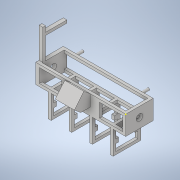
# Autodesk Inventor part: Diff housing
Saved by Autodesk Inventor 2021 (Build 250183000, 183)
## iProperties
Created: 2020-10-15
Part Number: Diff housing
Material: Generic
Document SubType Name: Modeling
Designer: nabee
Density: 1 g/cm^3
Appearance: Default
Author: nabee
Autodesk Inventor part; units mm, degrees
ref_plane "YZ Plane" through (0, 0, 0) normal (1, 0, 0) x (0, 1, 0)
ref_plane "XZ Plane" through (0, 0, 0) normal (0, 1, 0) x (-1, 0, 0)
sketch "Sketch1" plane through (0, 0, 0) normal (0, 0, 1) x (1, 0, 0)
  line L0 (0, 0) -> (500, 0)
  line L1 (500, 0) -> (500, 140)
  line L2 (500, 140) -> (0, 140)
  line L3 (0, 140) -> (0, 0)
  dimension "d0" = 140
  dimension "d1" = 500
  constraints: 8 end point, 2 parallel, 1 horizontal, 1 perpendicular
  measures "d0" distance of L2.end L0.start
  measures "d1" distance of L0.start L0.end
extrude "Extrusion1" add sketch "Sketch1" along normal blind 200
sketch "Sketch2" plane through (0, 140, 0) normal (0, 1, 0) x (1, 0, 0)
  line L0 (20, -20) -> (480, -20)
  line L1 (480, -20) -> (480, -180)
  line L2 (480, -180) -> (20, -180)
  line L3 (20, -180) -> (20, -20)
  line L4 (500, 0) -> (0, 0) projected
  line L5 (0, 0) -> (0, -200) projected
  line L6 (500, -200) -> (0, -200) projected
  line L7 (500, 0) -> (500, -200) projected
  dimension "d4" = 20
  dimension "d5" = 20
  dimension "d6" = 20
  dimension "d7" = 20
  constraints: 8 end point, 2 parallel, 1 horizontal, 1 perpendicular
  measures "d4" distance between parallel lines of L4 L0
  measures "d5" distance between parallel lines of L5 L3
  measures "d6" distance between parallel lines of L6 L2
  measures "d7" distance between parallel lines of L7 L1
extrude "Extrusion2" cut sketch "Sketch2" against normal blind 200 contours L0 L1 L2 L3
sketch "Sketch3" plane through (0, 0, 200) normal (0, 0, 1) x (1, 0, 0)
  line L0 (20, 120) -> (480, 120)
  line L1 (480, 120) -> (480, 20)
  line L2 (480, 20) -> (20, 20)
  line L3 (20, 20) -> (20, 120)
  line L4 (500, 140) -> (0, 140) projected
  line L5 (0, 140) -> (0, 0) projected
  line L6 (0, 0) -> (500, 0) projected
  line L7 (500, 0) -> (500, 140) projected
  dimension "d10" = 20
  dimension "d11" = 20
  dimension "d12" = 20
  dimension "d13" = 20
  constraints: 8 end point, 2 parallel, 1 horizontal, 1 perpendicular
  measures "d10" distance between parallel lines of L4 L0
  measures "d11" distance between parallel lines of L5 L3
  measures "d12" distance between parallel lines of L6 L2
  measures "d13" distance between parallel lines of L7 L1
extrude "Extrusion3" cut sketch "Sketch3" against normal blind 200 contours L0 L1 L2 L3
sketch "Sketch4" plane through (500, 0, 0) normal (1, 0, 0) x (0, 0, -1)
  line L0 (0, 140) -> (-200, 140) projected
  circle A0 centre (-100, 70) radius 23.813
  point P0 (0, 0)
  dimension "d16" = 47.626
  constraints: 1 centre point
  measures "d16" diameter of A0
extrude "Extrusion4" cut sketch "Sketch4" against normal blind 900
sketch "Sketch5" plane through (500, 0, 0) normal (1, 0, 0) x (0, 0, -1)
  line L0 (0, 140) -> (-200, 140) projected
  line L1 (-200, 140) -> (0, 140)
  line L2 (0, 140) -> (0, 0)
  line L3 (0, 0) -> (-200, 0)
  line L4 (-200, 0) -> (-200, 140)
  constraints: 8 end point, 2 parallel, 1 horizontal, 1 perpendicular
extrude "Extrusion5" add sketch "Sketch5" along normal blind 146.467
sketch "Sketch7" plane through (646.467, 0, 0) normal (1, 0, 0) x (0, 0, -1)
  circle A0 centre (-100, 70) radius 23.813 projected
  circle A1 centre (-100, 70) radius 23.813
  point P0 (0, 0)
  constraints: 1 centre point, 1 coincident
extrude "Extrusion6" cut sketch "Sketch7" against normal blind 146.467
sketch "Sketch8" plane through (0, 0, 200) normal (0, 0, 1) x (1, 0, 0)
  line L0 (20, 120) -> (480, 120) projected
  line L1 (480, 120) -> (626.467, 120)
  line L2 (626.467, 120) -> (626.467, 20)
  line L3 (626.467, 20) -> (480, 20)
  line L4 (480, 20) -> (480, 120)
  line L5 (646.467, 140) -> (646.467, 0) projected
  point P0 (0, 0)
  dimension "d27" = 20
  constraints: 8 end point, 2 parallel, 1 horizontal, 1 perpendicular
  measures "d27" distance between parallel lines of L5 L2
extrude "Extrusion7" cut sketch "Sketch8" against normal blind 600
sketch "Sketch9" plane through (0, 140, 200) normal (0, 1, 0) x (1, 0, 0)
  line L0 (480, 180) -> (20, 180) projected
  line L1 (480, 180) -> (626.467, 180)
  line L2 (626.467, 180) -> (626.467, 20)
  line L3 (626.467, 20) -> (480, 20)
  line L4 (480, 20) -> (480, 180)
  line L5 (646.467, 200) -> (646.467, 0) projected
  point P0 (0, 200)
  dimension "d30" = 20
  constraints: 8 end point, 2 parallel, 1 horizontal, 1 perpendicular
  measures "d30" distance between parallel lines of L5 L2
extrude "Extrusion8" cut sketch "Sketch9" against normal blind 600
sketch "Sketch10" plane through (646.467, 0, 0) normal (1, 0, 0) x (0, 0, -1)
  line L0 (-200, 140) -> (0, 140)
  line L1 (0, 140) -> (0, 0)
  line L2 (0, 0) -> (-200, 0)
  line L3 (-200, 0) -> (-200, 140)
  constraints: 8 end point, 2 parallel, 1 horizontal, 1 perpendicular
extrude "Extrusion9" add sketch "Sketch10" along normal blind 10
sketch "Sketch11" plane through (656.467, 0, 0) normal (1, 0, 0) x (0, 0, -1)
  line L0 (0, 140) -> (-200, 140) projected
  line L1 (0, 140) -> (0, 0) projected
  line L2 (-200, 140) -> (0, 140)
  line L3 (0, 140) -> (0, 0)
  line L4 (0, 0) -> (-200, 0)
  line L5 (-200, 0) -> (-200, 140)
  constraints: 8 end point, 2 parallel, 1 horizontal, 1 perpendicular
extrude "Extrusion10" cut sketch "Sketch11" against normal blind 3.764
sketch "Sketch12" plane through (652.703, 0, 0) normal (1, 0, 0) x (0, 0, -1)
  circle A0 centre (-100, 70) radius 23.813 projected
  circle A1 centre (-100, 70) radius 23.813
  point P0 (0, 0)
  constraints: 1 centre point, 1 coincident
extrude "Extrusion11" cut sketch "Sketch12" against normal blind 200
sketch "Sketch14" plane through (0, 0, 200) normal (0, 0, 1) x (1, 0, 0)
  line L0 (652.703, 140) -> (452.703, 140)
  line L1 (452.703, 140) -> (452.703, 0)
  line L2 (652.703, 0) -> (652.703, 140)
  line L3 (0, 0) -> (652.703, 0) projected
  line L4 (652.703, 0) -> (652.703, -140)
  line L5 (652.703, -140) -> (452.703, -140)
  line L6 (452.703, -140) -> (452.703, 0)
  dimension "d47" = 200
  dimension "d48" = 140
  constraints: 12 end point, 3 perpendicular, 1 horizontal, 1 parallel, 1 vertical
  measures "d47" distance of L0.start L0.end
  measures "d48" distance of L2.start L4.end
extrude "Extrusion13" add sketch "Sketch14" along normal blind 160
sketch "Sketch15" plane through (0, 0, 360) normal (0, 0, 1) x (1, 0, 0)
  line L0 (632.703, -120) -> (472.703, -120)
  line L1 (472.703, -120) -> (472.703, 120)
  line L2 (472.703, 120) -> (632.703, 120)
  line L3 (632.703, 120) -> (632.703, -120)
  line L4 (452.703, -140) -> (652.703, -140) projected
  line L5 (652.703, -140) -> (652.703, 140) projected
  line L6 (652.703, 140) -> (452.703, 140) projected
  line L7 (452.703, 140) -> (452.703, -140) projected
  point P0 (0, 0)
  dimension "d51" = 20
  dimension "d52" = 20
  dimension "d53" = 20
  dimension "d54" = 20
  constraints: 8 end point, 2 parallel, 1 horizontal, 1 perpendicular
  measures "d51" distance between parallel lines of L4 L0
  measures "d52" distance between parallel lines of L5 L3
  measures "d53" distance between parallel lines of L6 L2
  measures "d54" distance between parallel lines of L7 L1
extrude "Extrusion14" cut sketch "Sketch15" against normal blind 160 contours L0 L1 L2 L3
sketch "Sketch16" plane through (452.703, -140, 200) normal (-1, 0, 0) x (0, 0, 1)
  line L0 (140, 20) -> (20, 20)
  line L1 (20, 20) -> (20, 260)
  line L2 (20, 260) -> (140, 260)
  line L3 (140, 260) -> (140, 20)
  line L4 (0, 0) -> (160, 0) projected
  line L5 (160, 280) -> (160, 0) projected
  line L6 (0, 140) -> (0, 0) projected
  line L7 (0, 280) -> (160, 280) projected
  point P0 (-200, 140)
  dimension "d57" = 20
  dimension "d58" = 20
  dimension "d59" = 20
  dimension "d60" = 20
  constraints: 8 end point, 2 parallel, 1 horizontal, 1 perpendicular
  measures "d57" distance between parallel lines of L4 L0
  measures "d58" distance between parallel lines of L5 L3
  measures "d59" distance between parallel lines of L6 L1
  measures "d60" distance between parallel lines of L7 L2
extrude "Extrusion15" cut sketch "Sketch16" against normal blind 900
sketch "Sketch17" plane through (452.703, -140, 200) normal (0, -1, 0) x (1, 0, 0)
  line L0 (180, 160) -> (180, 140) projected
  line L1 (20, 20) -> (20, 0) projected
  line L2 (180, 140) -> (20, 140)
  line L3 (20, 140) -> (20, 20)
  line L4 (20, 20) -> (180, 20)
  line L5 (180, 20) -> (180, 140)
  point P0 (-452.703, -200)
  constraints: 8 end point, 2 parallel, 1 horizontal, 1 perpendicular
extrude "Extrusion16" cut sketch "Sketch17" against normal blind 900
sketch "Sketch18" plane through (452.703, -140, 200) normal (-1, 0, 0) x (0, 0, 1)
  line L0 (0, 280) -> (160, 280) projected
  line L1 (0, 0) -> (0, 140) projected
  line L2 (160, 280) -> (0, 280)
  line L3 (0, 280) -> (0, 0)
  line L4 (0, 0) -> (160, 0)
  line L5 (160, 0) -> (160, 280)
  point P0 (-200, 140)
  constraints: 8 end point, 2 parallel, 1 horizontal, 1 perpendicular
extrude "Extrusion17" cut sketch "Sketch18" against normal blind 10
sketch "Sketch19" plane through (472.703, -140, 340) normal (1, 0, 0) x (0, 0, -1)
  line L0 (140, 260) -> (140, 280) projected
  line L1 (-20, 0) -> (140, 0) projected
  line L2 (140, 280) -> (-20, 280)
  line L3 (-20, 280) -> (-20, 0)
  line L4 (-20, 0) -> (140, 0)
  line L5 (140, 0) -> (140, 280)
  point P0 (340, 140)
  constraints: 8 end point, 2 parallel, 1 horizontal, 1 perpendicular
extrude "Extrusion18" add sketch "Sketch19" along normal blind 10
sketch "Sketch20" plane through (472.703, -140, 340) normal (-1, 0, 0) x (0, 0, 1)
  line L0 (0, 20) -> (0, 260) projected
  line L1 (-120, 20) -> (-120, 260) projected
  line L2 (0, 20) -> (-120, 20)
  line L3 (-120, 20) -> (-120, 260)
  line L4 (-120, 260) -> (0, 260)
  line L5 (0, 260) -> (0, 20)
  point P0 (-340, 140)
  constraints: 8 end point, 2 parallel, 1 horizontal, 1 perpendicular
extrude "Extrusion19" cut sketch "Sketch20" against normal blind 10
sketch "Sketch23" plane through (0, 140, 200) normal (0, 1, 0) x (1, 0, 0)
  line L0 (652.703, 200) -> (652.703, 0) projected
  line L1 (652.703, 0) -> (0, 0)
  line L2 (0, 0) -> (0, 200)
  line L3 (0, 200) -> (652.703, 200)
  line L4 (652.703, 200) -> (652.703, 0)
  constraints: 8 end point, 2 parallel, 1 horizontal, 1 perpendicular
extrude "Extrusion21" add sketch "Sketch23" along normal blind 150
sketch "Sketch24" plane through (0, 290, 200) normal (0, 1, 0) x (1, 0, 0)
  line L0 (626.467, 20) -> (626.467, 180) projected
  line L1 (20, 180) -> (20, 20) projected
  line L2 (626.467, 20) -> (20, 20)
  line L3 (20, 20) -> (20, 180)
  line L4 (20, 180) -> (626.467, 180)
  line L5 (626.467, 180) -> (626.467, 20)
  point P0 (0, 200)
  constraints: 8 end point, 2 parallel, 1 horizontal, 1 perpendicular
extrude "Extrusion22" cut sketch "Sketch24" against normal blind 150
sketch "Sketch25" plane through (0, 0, 200) normal (0, 0, 1) x (1, 0, 0)
  point P0 (0, 0)
sketch "Sketch32" plane through (0, 0, 200) normal (0, 0, 1) x (1, 0, 0)
  line L0 (632.703, 140) -> (482.703, 140) projected
  line L1 (626.467, 290) -> (20, 290) projected
  line L2 (561.3515, 140) -> (541.3515, 140)
  line L3 (541.3515, 140) -> (541.3515, 290)
  line L4 (541.3515, 290) -> (561.3515, 290)
  line L5 (561.3515, 290) -> (561.3515, 140)
  line L6 (652.703, 140) -> (652.703, 290) projected
  line L7 (411.3515, 140) -> (391.3515, 140)
  line L8 (391.3515, 140) -> (391.3515, 290)
  line L9 (391.3515, 290) -> (411.3515, 290)
  line L10 (411.3515, 290) -> (411.3515, 140)
  line L11 (261.3515, 140) -> (241.3515, 140)
  line L12 (241.3515, 140) -> (241.3515, 290)
  line L13 (241.3515, 290) -> (261.3515, 290)
  line L14 (261.3515, 290) -> (261.3515, 140)
  line L15 (111.3515, 140) -> (91.3515, 140)
  line L16 (91.3515, 140) -> (91.3515, 290)
  line L17 (91.3515, 290) -> (111.3515, 290)
  line L18 (111.3515, 290) -> (111.3515, 140)
  point P0 (0, 0)
  dimension "d101" = 20
  dimension "d102" = 91.3515
  dimension "d103" = 20
  dimension "d104" = 130
  dimension "d105" = 20
  dimension "d106" = 130
  dimension "d107" = 20
  dimension "d108" = 130
  constraints: 32 end point, 8 parallel, 7 point on line, 4 horizontal, 4 perpendicular
  measures "d101" distance between parallel lines of L3 L5
  measures "d102" distance between parallel lines of L6 L5
  measures "d103" distance of L7.start L7.end
  measures "d104" distance between parallel lines of L3 L10
  measures "d105" distance of L11.start L11.end
  measures "d106" distance between parallel lines of L8 L14
  measures "d107" distance of L15.start L15.end
  measures "d108" distance between parallel lines of L12 L18
extrude "Extrusion26" add sketch "Sketch32" against normal up to surface (180 mm away)
sketch "Sketch33" plane through (0, 0, 200) normal (0, 0, 1) x (1, 0, 0)
  line L0 (652.703, 140) -> (462.703, 140) projected
  line L1 (0, 290) -> (652.703, 290) projected
  line L2 (652.703, 140) -> (561.3515, 140)
  line L3 (561.3515, 140) -> (561.3515, 290)
  line L4 (561.3515, 290) -> (652.703, 290)
  line L5 (652.703, 290) -> (652.703, 140)
  line L6 (541.3515, 290) -> (411.3515, 290)
  line L7 (411.3515, 290) -> (411.3515, 140)
  line L8 (411.3515, 140) -> (541.3515, 140)
  line L9 (541.3515, 140) -> (541.3515, 290)
  line L10 (391.3515, 140) -> (261.3515, 140)
  line L11 (261.3515, 140) -> (261.3515, 290)
  line L12 (261.3515, 290) -> (391.3515, 290)
  line L13 (391.3515, 290) -> (391.3515, 140)
  line L14 (241.3515, 140) -> (111.3515, 140)
  line L15 (111.3515, 140) -> (111.3515, 290)
  line L16 (111.3515, 290) -> (241.3515, 290)
  line L17 (241.3515, 290) -> (241.3515, 140)
  line L18 (91.3515, 140) -> (91.3515, 290) projected
  line L19 (91.3515, 140) -> (0, 140)
  line L20 (0, 140) -> (0, 290)
  line L21 (0, 290) -> (91.3515, 290)
  line L22 (91.3515, 290) -> (91.3515, 140)
  point P0 (0, 0)
  dimension "d111" = 91.3515
  dimension "d112" = 20
  dimension "d113" = 130
  dimension "d114" = 20
  dimension "d115" = 130
  dimension "d116" = 20
  dimension "d117" = 130
  constraints: 40 end point, 10 parallel, 6 point on line, 5 horizontal, 5 perpendicular
  measures "d111" distance of L3.end L4.end
  measures "d112" distance between parallel lines of L9 L3
  measures "d113" distance of L7.end L8.end
  measures "d114" distance between parallel lines of L13 L7
  measures "d115" distance of L10.start L10.end
  measures "d116" distance between parallel lines of L17 L11
  measures "d117" distance of L15.end L16.end
extrude "Extrusion27" cut sketch "Sketch33" against normal up to surface (200 mm away) contours L0 L3 L1 L5 | L0 L8 L7 L1 L9 | L1 L18 L19 L20 | L1 L17 L14 L15 | L1 L13 L10 L11
sketch "Sketch34" plane through (91.3515, 290, 0) normal (-1, 0, 0) x (0, 0, 1)
  line L0 (180, -119.896571) -> (20, -119.896571)
  line L1 (20, -119.896571) -> (20, -20)
  line L2 (20, -20) -> (180, -20)
  line L3 (180, -20) -> (180, -119.896571)
  line L4 (200, 0) -> (200, -150)
  line L5 (0, 0) -> (200, 0)
  line L6 (0, -150) -> (0, 0)
  point P0 (0, -290)
  dimension "d121" = 20
  dimension "d122" = 20
  dimension "d123" = 20
  constraints: 8 end point, 2 parallel, 1 horizontal, 1 perpendicular
  measures "d121" distance between parallel lines of L4 L3
  measures "d122" distance between parallel lines of L5 L2
  measures "d123" distance between parallel lines of L6 L1
extrude "Extrusion28" cut sketch "Sketch34" against normal blind 900
sketch "Sketch35" plane through (0, 290, 200) normal (0, 1, 0) x (1, 0, 0)
  line L0 (652.703, 0) -> (462.703, 0) projected
  line L1 (541.3515, 20) -> (541.3515, 180) projected
  line L2 (561.3515, 0) -> (541.3515, 0)
  line L3 (541.3515, 0) -> (541.3515, 200)
  line L4 (541.3515, 200) -> (561.3515, 200)
  line L5 (561.3515, 200) -> (561.3515, 0)
  line L6 (652.703, 0) -> (462.703, 0) projected
  line L7 (20, 200) -> (626.467, 200) projected
  line L8 (411.3515, 0) -> (391.3515, 0)
  line L9 (391.3515, 0) -> (391.3515, 200)
  line L10 (391.3515, 200) -> (411.3515, 200)
  line L11 (411.3515, 200) -> (411.3515, 0)
  line L12 (462.703, 0) -> (20, 0) projected
  line L13 (261.3515, 0) -> (241.3515, 0)
  line L14 (241.3515, 0) -> (241.3515, 200)
  line L15 (241.3515, 200) -> (261.3515, 200)
  line L16 (261.3515, 200) -> (261.3515, 0)
  line L17 (111.3515, 0) -> (91.3515, 0)
  line L18 (91.3515, 0) -> (91.3515, 200)
  line L19 (91.3515, 200) -> (111.3515, 200)
  line L20 (111.3515, 200) -> (111.3515, 0)
  point P0 (0, 200)
  point P1 (541.3515, 0)
  point P2 (111.3515, 0)
  point P3 (111.3515, 200)
  point P4 (91.3515, 0)
  point P5 (241.3515, 0)
  point P6 (411.3515, 200)
  dimension "d126" = 20
  dimension "d127" = 130
  dimension "d128" = 20
  dimension "d129" = 130
  dimension "d130" = 20
  constraints: 32 end point, 8 parallel, 5 point on line, 4 horizontal, 4 perpendicular
  measures "d126" distance of L8.start L8.end
  measures "d127" distance between parallel lines of L16 L9
  measures "d128" distance of L14.end L15.end
  measures "d129" distance between parallel lines of L14 L20
  measures "d130" distance between parallel lines of L18 L20
extrude "Extrusion29" add sketch "Sketch35" along normal blind 20 contours L8 L9 L7 L11 | L12 L14 L7 L16 | L12 L18 L7 L20
sketch "Sketch36" plane through (91.3515, 140, 20) normal (-1, 0, 0) x (0, 0, 1)
  line L0 (160, 130) -> (0, 130) projected
  line L1 (160, 130) -> (0, 130)
  line L2 (0, 130) -> (0, 150)
  line L3 (0, 150) -> (160, 150)
  line L4 (160, 150) -> (160, 130)
  line L5 (-20, 170) -> (180, 170) projected
  point P0 (-20, -140)
  point P1 (0, 130)
  dimension "d134" = 20
  constraints: 8 end point, 2 parallel, 1 horizontal, 1 perpendicular
  measures "d134" distance between parallel lines of L5 L3
extrude "Extrusion30" cut sketch "Sketch36" against normal up to surface (470 mm away)
sketch "Sketch37" plane through (91.3515, 140, 20) normal (-1, 0, 0) x (0, 0, 1)
  line L0 (160, 30.103429) -> (0, 30.103429)
  line L1 (0, 30.103429) -> (0, 20.103429)
  line L2 (0, 20.103429) -> (160, 20.103429)
  line L3 (160, 20.103429) -> (160, 30.103429)
  point P0 (-20, -140)
  dimension "d137" = 10
  constraints: 8 end point, 2 parallel, 1 horizontal, 1 perpendicular
  measures "d137" distance of L0.end L1.end
extrude "Extrusion31" cut sketch "Sketch37" against normal up to surface (470 mm away)
sketch "Sketch39" plane through (541.3515, 290, 20) normal (0, 0, 1) x (1, 0, 0)
  line L0 (20, -80) -> (0, -80)
  line L1 (0, -80) -> (0, -50)
  line L2 (0, -50) -> (20, -50)
  line L3 (20, -50) -> (20, -80)
  line L4 (-130, -80) -> (-150, -80)
  line L5 (-150, -80) -> (-150, -50)
  line L6 (-150, -50) -> (-130, -50)
  line L7 (-130, -50) -> (-130, -80)
  line L8 (-280, -80) -> (-300, -80)
  line L9 (-300, -80) -> (-300, -50)
  line L10 (-300, -50) -> (-280, -50)
  line L11 (-280, -50) -> (-280, -80)
  line L12 (-430, -129.896571) -> (-430, 0)
  line L13 (-450, -129.896571) -> (-450, 0)
  line L14 (-430, -80) -> (-450, -80)
  line L15 (-450, -80) -> (-450, -50)
  line L16 (-450, -50) -> (-430, -50)
  line L17 (-430, -50) -> (-430, -80)
  line L18 (111.3515, -150) -> (-78.6485, -150)
  line L19 (0, 20) -> (20, 20)
  line L20 (20, -150) -> (-78.6485, -150)
  line L21 (-150, 20) -> (-130, 20)
  line L22 (-300, 20) -> (-280, 20)
  line L23 (-450, 20) -> (-430, 20)
  point P0 (-541.3515, -290)
  point P1 (-130, -150)
  dimension "d140" = 70
  dimension "d141" = 70
  dimension "d142" = 70
  dimension "d143" = 70
  dimension "d144" = 70
  dimension "d145" = 70
  constraints: 32 end point, 8 parallel, 4 horizontal, 4 perpendicular, 4 point on line
  measures "d140" distance between parallel lines of L18 L0
  measures "d141" distance between parallel lines of L19 L2
  measures "d142" distance between parallel lines of L20 L4
  measures "d143" distance between parallel lines of L21 L6
  measures "d144" distance between parallel lines of L22 L10
  measures "d145" distance between parallel lines of L23 L16
extrude "Extrusion32" add sketch "Sketch39" along normal blind 20
sketch "Sketch40" plane through (411.3515, 290, 180) normal (0, 0, -1) x (-1, 0, 0)
  line L0 (320, 0) -> (320, -129.896571)
  line L1 (320, -80) -> (300, -80)
  line L2 (300, -80) -> (300, -50)
  line L3 (300, -50) -> (320, -50)
  line L4 (320, -50) -> (320, -80)
  line L5 (411.3515, -150) -> (320, -150)
  line L6 (300, 20) -> (320, 20)
  line L7 (170, -129.896571) -> (170, -80)
  line L8 (150, -129.896571) -> (150, 0)
  line L9 (170, -80) -> (150, -80)
  line L10 (150, -80) -> (150, -50)
  line L11 (150, -50) -> (170, -50)
  line L12 (170, -50) -> (170, -80)
  line L13 (20, -129.896571) -> (20, -80)
  line L14 (0, 20) -> (0, -150)
  line L15 (20, -80) -> (0, -80)
  line L16 (0, -80) -> (0, -50)
  line L17 (0, -50) -> (20, -50)
  line L18 (20, -50) -> (20, -80)
  line L19 (-130, 0) -> (-130, -150)
  line L20 (-150, 0) -> (-150, -150)
  line L21 (-130, -80) -> (-150, -80)
  line L22 (-150, -80) -> (-150, -50)
  line L23 (-150, -50) -> (-130, -50)
  line L24 (-130, -50) -> (-130, -80)
  point P0 (411.3515, -290)
  point P1 (-130, 20)
  point P2 (-150, 20)
  point P3 (-130, -50)
  point P4 (-150, -80)
  point P5 (0, -80)
  dimension "d148" = 70
  dimension "d149" = 70
  constraints: 32 end point, 8 parallel, 8 point on line, 4 horizontal, 4 perpendicular
  measures "d148" distance between parallel lines of L5 L1
  measures "d149" distance between parallel lines of L6 L3
extrude "Extrusion33" add sketch "Sketch40" along normal blind 20
sketch "Sketch41" plane through (241.3515, 140, 180) normal (0, -1, 0) x (1, 0, 0)
  line L0 (320, 0) -> (320, -160)
  line L1 (300, 0) -> (300, -160)
  line L2 (320, -160) -> (300, -160)
  line L3 (300, -160) -> (300, 0)
  line L4 (300, 0) -> (320, 0)
  line L5 (320, 0) -> (320, -160)
  line L6 (300, -160) -> (170, -160)
  line L7 (150, -180) -> (150, 20)
  line L8 (170, -160) -> (150, -160)
  line L9 (150, -160) -> (150, 0)
  line L10 (150, 0) -> (170, 0)
  line L11 (170, 0) -> (170, -160)
  line L12 (150, -160) -> (20, -160)
  line L13 (20, -160) -> (0.004718, -160)
  line L14 (0.004718, -160) -> (0.004718, 0)
  line L15 (0.004718, 0) -> (20, 0)
  line L16 (20, 0) -> (20, -160)
  line L17 (0, -160) -> (-130, -160)
  line L18 (-150, -160) -> (-150, 0)
  line L19 (-130, -160) -> (-150, -160)
  line L20 (-150, -160) -> (-150, 0)
  line L21 (-150, 0) -> (-130, 0)
  line L22 (-130, 0) -> (-130, -160)
  point P0 (-241.3515, -180)
  constraints: 32 end point, 8 parallel, 4 horizontal, 4 perpendicular, 3 point on line
extrude "Extrusion34" add sketch "Sketch41" along normal blind 20
sketch "Sketch42" plane through (0, 0, 200) normal (0, 0, 1) x (1, 0, 0)
  line L0 (626.467, 120) -> (20, 120) projected
  line L1 (626.467, 0) -> (20, 0) projected
  line L2 (462.703, 120) -> (190, 120)
  line L3 (190, 120) -> (190, 0)
  line L4 (190, 0) -> (462.703, 0)
  line L5 (462.703, 0) -> (462.703, 120)
  line L6 (652.703, -140) -> (652.703, 140) projected
  line L7 (0, 0) -> (0, 140) projected
  line L8 (462.703, 140) -> (462.703, -140) projected
  point P0 (541.3515, 120)
  point P1 (411.3515, 120)
  point P2 (462.703, 0)
  dimension "d155" = 190
  dimension "d158" = 0
  constraints: 8 end point, 2 parallel, 2 point on line, 1 horizontal, 1 perpendicular
  measures "d155" distance between parallel lines of L7 L3
  measures "d158" distance between parallel lines of L8 L5
extrude "Extrusion35" add sketch "Sketch42" against normal blind 20
sketch "Sketch43" plane through (0, 0, 360) normal (0, 0, 1) x (1, 0, 0)
  line L0 (462.703, -140) -> (652.703, -140) projected
  line L1 (411.3515, 140) -> (541.3515, 140) projected
  line L2 (652.703, -140) -> (462.703, -140)
  line L3 (462.703, -140) -> (462.703, 140)
  line L4 (462.703, 140) -> (652.703, 140)
  line L5 (652.703, 140) -> (652.703, -140)
  point P0 (0, 0)
  dimension "d159" = 190
  constraints: 8 end point, 2 parallel, 1 horizontal, 1 perpendicular, 1 point on line
  measures "d159" distance of L3.end L4.end
extrude "Extrusion36" cut sketch "Sketch43" against normal up to surface (160 mm away)
sketch "Sketch44" plane through (0, 0, 200) normal (0, 0, 1) x (1, 0, 0)
  line L0 (241.3515, 140) -> (111.3515, 140) projected
  line L1 (442.703, 0) -> (210, 0)
  line L2 (210, 0) -> (210, 140)
  line L3 (210, 140) -> (442.703, 140)
  line L4 (442.703, 140) -> (442.703, 0)
  line L5 (462.703, 20) -> (462.703, 120) projected
  line L6 (190, 120) -> (190, 20) projected
  point P0 (0, 0)
  dimension "d162" = 20
  dimension "d163" = 20
  constraints: 8 end point, 2 parallel, 1 horizontal, 1 perpendicular, 1 point on line
  measures "d162" distance between parallel lines of L5 L4
  measures "d163" distance between parallel lines of L6 L2
ref_plane "Work Plane2" through (0, 0, 270) normal (0, 0, 1) x (1, 0, 0)
sketch "Sketch45" plane through (0, 0, 270) normal (0, 0, 1) x (1, 0, 0)
  line L0 (652.703, 140) -> (462.703, 140) projected
  line L1 (442.703, 140) -> (210, 140)
  line L2 (210, 140) -> (210, 85)
  line L3 (210, 85) -> (442.703, 85)
  line L4 (442.703, 85) -> (442.703, 140)
  line L5 (652.703, 140) -> (652.703, 0) projected
  point P0 (0, 0)
  point P1 (411.3515, 140)
  point P2 (541.3515, 140)
  dimension "d165" = 232.703
  dimension "d166" = 210
  dimension "d171" = 55
  constraints: 8 end point, 2 parallel, 1 horizontal, 1 perpendicular, 1 point on line
  measures "d165" distance of L1.start L1.end
  measures "d166" distance between parallel lines of L5 L4
  measures "d171" distance of L1.end L2.end
sketch "Sketch44 outline for Loft1" plane through (0, 0, 200) normal (0, 0, 1) x (1, 0, 0)
  line L0 (442.703, 0) -> (210, 0)
  line L1 (210, 0) -> (210, 140)
  line L2 (210, 140) -> (442.703, 140)
  line L3 (442.703, 140) -> (442.703, 0)
sketch "Sketch45 outline for Loft1" plane through (0, 0, 270) normal (0, 0, 1) x (1, 0, 0)
  line L0 (442.703, 85) -> (442.703, 140)
  line L1 (210, 85) -> (442.703, 85)
  line L2 (210, 140) -> (210, 85)
  line L3 (442.703, 140) -> (210, 140)
loft "Loft1" add profiles "Sketch44 outline for Loft1", "Sketch45 outline for Loft1"
sketch "Sketch46" plane through (210, 0, 200) normal (0, -0.6357073, 0.7719302) x (1, 0, 0)
  line L0 (232.703, 0) -> (442.703, 0)
  line L1 (0, 108.070233) -> (-98.6485, 108.070233)
  line L2 (232.703, 0) -> (0, 0)
  line L3 (0, 0) -> (0, 108.070233)
  line L4 (0, 108.070233) -> (232.703, 108.070233)
  line L5 (232.703, 108.070233) -> (232.703, 0)
  point P0 (-210, -127.141451)
  constraints: 8 end point, 2 parallel, 1 horizontal, 1 perpendicular
extrude "Extrusion37" add sketch "Sketch46" along normal blind 60
sketch "Sketch47" plane through (210, 85, 270) normal (0, 0, 1) x (1, 0, 0)
  line L0 (0, -1.57732) -> (232.703, -1.57732)
  line L1 (-98.6485, 55) -> (31.3515, 55)
  line L2 (232.703, -1.57732) -> (-0.004, -1.57732)
  line L3 (-0.004, -1.57732) -> (-0.004, 55)
  line L4 (-0.004, 55) -> (232.703, 55)
  line L5 (232.703, 55) -> (232.703, -1.57732)
  point P0 (-210, -85)
  point P1 (31.3515, 55)
  dimension "d174" = 232.707
  constraints: 8 end point, 2 parallel, 1 horizontal, 1 perpendicular, 1 point on line
  measures "d174" distance of L3.end L4.end
extrude "Extrusion38" cut sketch "Sketch47" against normal up to surface (70 mm away)
sketch "Sketch48" plane through (210, -38.142435, 246.315814) normal (0, -0.6357073, 0.7719302) x (1, 0, 0)
  line L0 (0, 0) -> (232.703, 0)
  line L1 (232.703, 108.070233) -> (202.703, 108.070233)
  line L2 (202.703, 108.070233) -> (202.703, 0)
  line L3 (202.703, 0) -> (232.703, 0)
  line L4 (232.703, 0) -> (232.703, 108.070233)
  line L5 (0, 0) -> (30, 0)
  line L6 (30, 0) -> (30, 108.070233)
  line L7 (30, 108.070233) -> (0, 108.070233)
  line L8 (0, 108.070233) -> (0, 0)
  point P0 (-210, -127.141451)
  dimension "d177" = 30
  dimension "d178" = 30
  constraints: 16 end point, 4 parallel, 2 horizontal, 2 perpendicular, 2 point on line
  measures "d177" distance of L7.end L6.end
  measures "d178" distance of L1.start L1.end
extrude "Extrusion39" cut sketch "Sketch48" against normal up to surface surface through (250, 70, 200) normal (0, 0, 1)
sketch "Sketch49" plane through (0, 0, 0) normal (0, 0, -1) x (-1, 0, 0)
  circle A0 centre (-561.203, 10) radius 9
  line L0 (-652.703, 0) -> (-652.703, 140) projected
  line L1 (-20, 20) -> (-626.467, 20) projected
  circle A1 centre (-85, 10) radius 9
  line L2 (0, 0) -> (0, 140) projected
  line L3 (0, 0) -> (-652.703, 0) projected
  dimension "d181" = 18
  dimension "d182" = 91.5
  dimension "d183" = 10
  dimension "d184" = 18
  dimension "d185" = 85
  dimension "d186" = 10
  constraints: 2 centre point
  measures "d181" diameter of A0
  measures "d182" distance from line of L0 A0.centre
  measures "d183" distance from line of L1 A0.centre
  measures "d184" diameter of A1
  measures "d185" distance from line of L2 A1.centre
  measures "d186" distance from line of L3 A1.centre
extrude "Extrusion40" add sketch "Sketch49" along normal blind 50
sketch "Sketch50" plane through (0, 290, 200) normal (0, 1, 0) x (1, 0, 0)
  line L0 (561.3515, 200) -> (541.3515, 200) projected
  line L1 (561.3515, 180) -> (561.3515, 200) projected
  line L2 (541.3515, 200) -> (561.3515, 200)
  line L3 (561.3515, 200) -> (561.3515, 180)
  line L4 (561.3515, 180) -> (541.3515, 180)
  line L5 (541.3515, 180) -> (541.3515, 200)
  line L6 (626.467, 0) -> (462.703, 0) projected
  line L7 (561.3515, 0) -> (561.3515, 20) projected
  line L8 (541.3515, 0) -> (561.3515, 0)
  line L9 (561.3515, 0) -> (561.3515, 20)
  line L10 (561.3515, 20) -> (541.3515, 20)
  line L11 (541.3515, 20) -> (541.3515, 0)
  point P0 (0, 200)
  constraints: 16 end point, 4 parallel, 2 horizontal, 2 perpendicular, 2 point on line
extrude "Extrusion41" add sketch "Sketch50" along normal up to surface (20 mm away)
sketch "Sketch51" plane through (561.3515, 240, 180) normal (0, 0, -1) x (-1, 0, 0)
  line L0 (20, 70) -> (0, 70) projected
  line L1 (0, 0) -> (0, 70) projected
  line L2 (20, 70) -> (0, 70)
  line L3 (0, 70) -> (0, 50)
  line L4 (0, 50) -> (20, 50)
  line L5 (20, 50) -> (20, 70)
  point P0 (561.3515, -240)
  dimension "d191" = 20
  constraints: 8 end point, 2 parallel, 1 horizontal, 1 perpendicular, 1 point on line
  measures "d191" distance of L4.end L0.start
extrude "Extrusion42" add sketch "Sketch51" along normal up to surface (180 mm away)
sketch "Sketch53" plane through (0, 0, 0) normal (0, -1, 0) x (1, 0, 0)
  line L0 (626.467, 180) -> (626.467, 20)
  line L1 (653.101277, 155) -> (626.467, 155)
  line L2 (626.467, 155) -> (626.467, 175)
  line L3 (626.467, 175) -> (653.101277, 175)
  line L4 (653.101277, 175) -> (653.101277, 155)
  line L5 (412.703, 200) -> (652.703, 200)
  point P0 (0, 0)
  dimension "d199" = 20
  dimension "d200" = 45
  constraints: 8 end point, 2 parallel, 1 horizontal, 1 perpendicular, 1 point on line
  measures "d199" distance of L3.end L1.start
  measures "d200" distance between parallel lines of L5 L1
extrude "Extrusion44" add sketch "Sketch53" along normal blind 179
sketch "Sketch55" plane through (652.703, 0, 155) normal (0, 0, -1) x (-1, 0, 0)
  line L0 (-0.398277, 0) -> (-0.398277, -179)
  line L1 (26.236, -179) -> (-0.398277, -179)
  line L2 (-0.398277, -179) -> (-0.398277, -159)
  line L3 (-0.398277, -159) -> (26.236, -159)
  line L4 (26.236, -159) -> (26.236, -179)
  point P0 (652.703, 0)
  dimension "d203" = 20
  constraints: 8 end point, 2 parallel, 1 horizontal, 1 perpendicular, 1 point on line
  measures "d203" distance of L3.end L1.start
extrude "Extrusion45" add sketch "Sketch55" along normal blind 155.004
sketch "Sketch56" plane through (0, -179, 0) normal (0, -1, 0) x (1, 0, 0)
  line L0 (653.101277, 175) -> (626.467, 175)
  line L1 (652.703, 155) -> (653.101277, 155)
  line L2 (626.467, 175) -> (653.101277, 175)
  line L3 (653.101277, 175) -> (653.101277, 155)
  line L4 (653.101277, 155) -> (626.467, 155)
  line L5 (626.467, 155) -> (626.467, 175)
  point P0 (0, 0)
  constraints: 8 end point, 2 parallel, 1 horizontal, 1 perpendicular
extrude "Extrusion47" add sketch "Sketch56" along normal blind 41.015
sketch "Sketch57" plane through (210, -38.142435, 246.315814) normal (0, -0.6357073, 0.7719302) x (1, 0, 0)
  line L0 (202.703, 0) -> (442.703, 0)
  line L1 (202.703, 108.070233) -> (30, 108.070233)
  line L2 (202.703, 0) -> (185.703, 0)
  line L3 (185.703, 0) -> (185.703, 108.070233)
  line L4 (185.703, 108.070233) -> (202.703, 108.070233)
  line L5 (202.703, 108.070233) -> (202.703, 0)
  line L6 (-210, 0) -> (30, 0)
  line L7 (30, 0) -> (47, 0)
  line L8 (47, 0) -> (47, 108.070233)
  line L9 (47, 108.070233) -> (30, 108.070233)
  line L10 (30, 108.070233) -> (30, 0)
  point P0 (-210, -127.141451)
  point P1 (47, 108.070233)
  point P2 (30, 108.070233)
  dimension "d210" = 17
  dimension "d211" = 17
  constraints: 16 end point, 4 parallel, 2 horizontal, 2 perpendicular, 2 point on line
  measures "d210" distance of L3.end L4.end
  measures "d211" distance of L9.end L8.end
extrude "Extrusion48" cut sketch "Sketch57" against normal up to surface surface through (250, 70, 200) normal (0, 0, 1)
body "Solid1"
